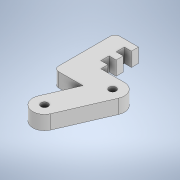
# Autodesk Inventor part: Chwytak wersja 3 - baza
Saved by Autodesk Inventor 2020 (Build 240168000, 168)
## iProperties
Created: 2019-07-08
Part Number: Chwytak wersja 3 - baza
Material: Generic
Document SubType Name: Modeling
Designer: WIN10
Density: 1 g/cm^3
Appearance: Default
Author: WIN10
Autodesk Inventor part; units mm, degrees
ref_plane "YZ Plane" through (0, 0, 0) normal (1, 0, 0) x (0, 1, 0)
ref_plane "XZ Plane" through (0, 0, 0) normal (0, 1, 0) x (-1, 0, 0)
ref_plane "XY Plane" through (0, 0, 0) normal (0, 0, 1) x (1, 0, 0)
sketch "Szkic1" plane through (0, 0, 0) normal (0, 1, 0) x (-1, 0, 0)
  arc A0 (13.307, 18.2188) -> (4.1253, 22.1807) centre (8.7161, 20.1997) ccw
  line L0 (4.1253, 22.1807) -> (-4.5909, 1.9809)
  line L1 (13.307, 18.2188) -> (7.6031, 5)
  arc A1 (-4.5909, 1.9809) -> (0, -5) centre (0, 0) ccw
  line L2 (8, -5) -> (10.5, -5) construction
  line L3 (10, -19) -> (10, -20)
  line L4 (10, -20) -> (10, -21)
  line L5 (10, -7) -> (10, -5)
  line L6 (10, -12) -> (10, -14)
  line L7 (10, -14) -> (10, -14.5)
  line L8 (20, -21) -> (10, -21)
  line L9 (13, -18) -> (10, -18)
  line L10 (10, -18) -> (10, -19)
  line L11 (10, -7) -> (10, -8)
  line L12 (10, -8) -> (13, -8)
  line L13 (13, -11.5) -> (10, -11.5)
  line L14 (10, -11.5) -> (10, -12)
  line L15 (13, -14.5) -> (10, -14.5)
  line L16 (10, -18) -> (13, -18)
  line L17 (13, -8) -> (13, -11.5)
  line L18 (13, -14.5) -> (13, -18)
  line L19 (18, 5) -> (20, 5)
  line L20 (20, 5) -> (20, -21)
  line L21 (20, -21) -> (18, -21)
  line L22 (0, -5) -> (10, -5)
  line L23 (18, 5) -> (7.6031, 5)
  arc A2 (13.307, 18.2188) -> (4.1253, 22.1807) centre (8.7161, 20.1997) ccw
  constraints: 48 end point, 6 point on circle, 5 horizontal, 5 perpendicular, 3 centre point, 3 tangent, 2 vertical, 1 collinear
extrude "Wyciągnięcie proste6" add sketch "Szkic1" along normal mid plane 6
fillet "Zaokrąglenie3" radius 2 2 edges at (-20, 0, -21) (-20, 0, 5)
fillet_without_effect "Fillet4"
sketch "Sketch8" plane through (0, 3, 0) normal (0, 1, 0) x (1, 0, 0)
  point P0 (0, 0)
  point P1 (0, 0)
  constraints: 1 coincident
hole "Hole1" at (0, 3, 0) direction (0, -1, 0) diameter 3 end through all
sketch "Sketch9" plane through (0, 3, 0) normal (0, 1, 0) x (1, 0, 0)
  arc A0 (-13.307, -18.2188) -> (-4.1253, -22.1807) centre (-8.7161, -20.1997) ccw projected
  point P0 (0, 0)
  constraints: 1 coincident
hole "Hole2" at (-8.7161, 3, 20.1997) direction (0, -1, 0) diameter 3 end through all
